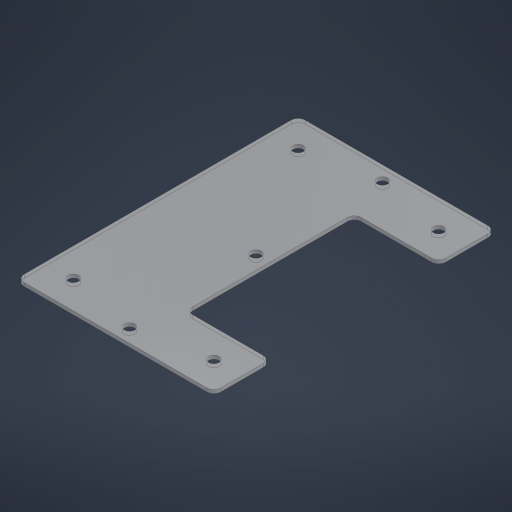
# Autodesk Inventor part: triball holder
Saved by Autodesk Inventor 2024 (Build 280153000, 153)
## iProperties
Created: 2023-12-13
Part Number: triball holder
Material: Generic
Document SubType Name: Modeling
Designer: macbook
Density: 1 g/cm^3
Appearance: Polycarbonate - Clear(1)
Author: macbook
Autodesk Inventor part; units mm, degrees
ref_plane "YZ Plane" through (0, 0, 0) normal (1, 0, 0) x (0, 1, 0)
ref_plane "XZ Plane" through (0, 0, 0) normal (0, 1, 0) x (-1, 0, 0)
ref_plane "XY Plane" through (0, 0, 0) normal (0, 0, 1) x (1, 0, 0)
sketch "Sketch1" plane through (0, 0, 0) normal (0, 1, 0) x (-1, 0, 0)
  line L0 (3.175, 0) -> (85.725, 0)
  line L1 (88.9, -3.175) -> (88.9, -123.825)
  line L2 (85.725, -127) -> (3.175, -127)
  line L3 (0, -123.825) -> (0, -104.775)
  line L4 (3.175, -101.6) -> (34.925, -101.6)
  line L5 (0, -3.175) -> (0, -22.225)
  line L6 (3.175, -25.4) -> (34.925, -25.4)
  line L7 (38.1, -28.575) -> (38.1, -98.425)
  arc A0 (88.9, -3.175) -> (85.725, 0) centre (85.725, -3.175) ccw
  arc A1 (85.725, -127) -> (88.9, -123.825) centre (85.725, -123.825) ccw
  arc A2 (0, -123.825) -> (3.175, -127) centre (3.175, -123.825) ccw
  arc A3 (3.175, -101.6) -> (0, -104.775) centre (3.175, -104.775) ccw
  arc A4 (34.925, -101.6) -> (38.1, -98.425) centre (34.925, -98.425) ccw
  arc A5 (3.175, 0) -> (0, -3.175) centre (3.175, -3.175) ccw
  arc A6 (0, -22.225) -> (3.175, -25.4) centre (3.175, -22.225) ccw
  arc A7 (38.1, -28.575) -> (34.925, -25.4) centre (34.925, -28.575) ccw
  line L8 (0, 0) -> (0, -12.7)
  line L9 (0, 0) -> (0, -12.7)
  line L10 (0, -12.7) -> (12.7, -12.7)
  line L11 (12.7, -12.7) -> (76.2, -12.7)
  line L12 (0, -114.3) -> (12.7, -114.3)
  line L13 (12.7, -114.3) -> (76.2, -114.3)
  line L14 (76.2, -12.7) -> (44.45, -12.7)
  line L15 (44.45, -12.7) -> (44.45, -6.35)
  line L16 (76.2, -114.3) -> (44.45, -114.3)
  line L17 (44.45, -114.3) -> (44.45, -120.65)
  line L18 (44.45, -12.7) -> (44.45, -114.3)
  line L19 (44.45, -63.5) -> (52.1099, -63.5)
  point P0 (88.9, 0)
  point P1 (88.9, -127)
  point P2 (0, -127)
  point P3 (0, -101.6)
  point P4 (38.1, -101.6)
  point P5 (0, -25.4)
  dimension "d0" = 88.9
  dimension "d1" = 127
  dimension "d2" = 25.4
  dimension "d3" = 38.1
  dimension "d4" = 25.4
  dimension "d5" = 3.175
  dimension "d8" = 12.7
  dimension "d10" = 63.5
  dimension "d11" = 31.75
  dimension "d12" = 6.35
  constraints: 40 end point, 16 point on circle, 16 tangent, 15 point on line, 8 centre point, 8 perpendicular, 7 equal radius, 5 horizontal, 5 midpoint, 2 collinear, 1 parallel, 1 vertical
  measures "d0" distance of L8.start point (88.9, 0)
  measures "d1" distance of point (88.9, 0) point (88.9, -127)
  measures "d2" distance of point (0, -127) point (0, -101.6)
  measures "d3" distance of point (0, -101.6) point (38.1, -101.6)
  measures "d4" distance of L8.start point (0, -25.4)
  measures "d5" radius of A0
  measures "d8" distance of L8.end L10.end
  measures "d10" distance of L10.end L11.end
  measures "d11" distance of L11.end L14.end
  measures "d12" distance of L16.end L17.end
extrude "Extrusion1" add sketch "Sketch1" along normal blind 1.5875
hole "Hole1" at (-76.2, 0, -12.7) at (-44.45, 0, -6.35) at (-12.7, 0, -12.7) at (-12.7, 0, -114.3) at (-44.45, 0, -120.65) at (-76.2, 0, -114.3) at (-44.45, 0, -63.5) direction (0, 1, 0) diameter 4.7625 end through all
body "Solid1"
